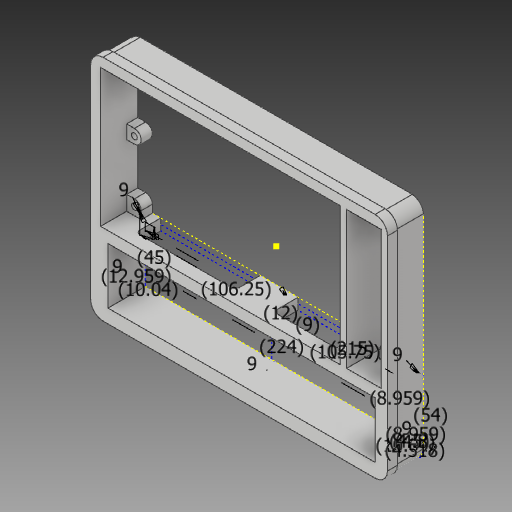
# Autodesk Inventor part: CyberDeckCover3
Saved by Autodesk Inventor 2019.4 (Build 234330000, 330)
## iProperties
Created: 2020-07-12
Part Number: CyberDeckCover3
Material: Generic
Document SubType Name: Modeling
Designer: Briti
Density: 1 g/cm^3
Appearance: Default
Author: Briti
Autodesk Inventor part; units mm, degrees
ref_plane "YZ Plane" through (0, 0, 0) normal (1, 0, 0) x (0, 1, 0)
ref_plane "XZ Plane" through (0, 0, 0) normal (0, 1, 0) x (-1, 0, 0)
ref_plane "XY Plane" through (0, 0, 0) normal (0, 0, 1) x (1, 0, 0)
sketch "Sketch1" plane through (0, 0, 0) normal (0, 0, 1) x (1, 0, 0)
  line L0 (-119.459, -91.9) -> (119.459, -91.9)
  line L1 (119.459, -91.9) -> (119.459, 91.9)
  line L2 (119.459, 91.9) -> (-119.459, 91.9)
  line L3 (-119.459, 91.9) -> (-119.459, -91.9)
  line L4 (-119.459, -91.9) -> (119.459, 91.9) construction
  line L5 (119.459, -91.9) -> (-119.459, 91.9) construction
  point P0 (0, 0)
  dimension "d0" = 238.918
  dimension "d1" = 183.8
  constraints: 12 end point, 2 midpoint, 2 parallel, 1 horizontal, 1 perpendicular
  measures "d0" distance of L2.end L1.end
  measures "d1" distance of L0.end L1.end
extrude "Extrusion1" add sketch "Sketch1" along normal blind 30
sketch "Sketch2" plane through (0, 0, 30) normal (0, 0, 1) x (1, 0, 0)
  arc A0 (-109.459, 91.9) -> (-119.459, 81.9) centre (-109.459, 81.9) ccw
  line L0 (119.459, 91.9) -> (-119.459, 91.9) projected
  line L1 (-119.459, 91.9) -> (-119.459, -91.9) projected
  line L2 (-119.459, 81.9) -> (-119.459, 91.9)
  line L3 (-109.459, 91.9) -> (-119.459, 91.9)
  arc A1 (-119.459, -81.9) -> (-109.459, -91.9) centre (-109.459, -81.9) ccw
  line L4 (-119.459, -91.9) -> (119.459, -91.9) projected
  line L5 (-119.459, -81.9) -> (-119.459, -91.9)
  line L6 (-109.459, -91.9) -> (-119.459, -91.9)
  arc A2 (109.459, -91.9) -> (119.459, -81.9) centre (109.459, -81.9) ccw
  line L7 (119.459, -91.9) -> (119.459, 91.9) projected
  line L8 (109.459, -91.9) -> (119.459, -91.9)
  line L9 (119.459, -81.9) -> (119.459, -91.9)
  arc A3 (119.459, 81.9) -> (109.459, 91.9) centre (109.459, 81.9) ccw
  line L10 (109.459, 91.9) -> (119.459, 91.9)
  line L11 (119.459, 81.9) -> (119.459, 91.9)
  point P0 (0, 0)
  dimension "d4" = 20
  dimension "d5" = 20
  dimension "d6" = 20
  dimension "d7" = 20
  constraints: 16 end point, 16 tangent, 8 point on circle, 8 point on line, 7 collinear, 4 centre point, 1 perpendicular
  measures "d4" diameter of A0
  measures "d5" diameter of A1
  measures "d6" diameter of A2
  measures "d7" diameter of A3
extrude "Extrusion2" add sketch "Sketch2" along normal blind 1 contours L0 A3 L7 A2 L4 A1 L1 A0
sketch "Sketch3" plane through (0, 0, 30) normal (0, 0, 1) x (1, 0, 0)
  line L0 (-119.459, -81.9) -> (-119.459, -91.9) projected
  arc A0 (-119.459, -81.9) -> (-109.459, -91.9) centre (-109.459, -81.9) ccw projected
  arc A1 (-119.459, -81.9) -> (-109.459, -91.9) centre (-109.459, -81.9) ccw
  line L1 (-119.459, -81.9) -> (-119.459, -91.9)
  line L2 (-119.459, -91.9) -> (-109.459, -91.9) projected
  line L3 (-109.459, -91.9) -> (-119.459, -91.9)
  arc A2 (-109.459, 91.9) -> (-119.459, 81.9) centre (-109.459, 81.9) ccw projected
  line L4 (-119.459, 81.9) -> (-119.459, -81.9) projected
  arc A3 (-109.459, 91.9) -> (-119.459, 81.9) centre (-109.459, 81.9) ccw
  line L5 (-119.459, 91.9) -> (-119.459, -91.9) projected
  line L6 (-119.459, 81.9) -> (-119.459, 91.9)
  line L7 (-119.459, 91.9) -> (-109.459, 91.9)
  arc A4 (119.459, 81.9) -> (109.459, 91.9) centre (109.459, 81.9) ccw projected
  arc A5 (119.459, 81.9) -> (109.459, 91.9) centre (109.459, 81.9) ccw
  line L8 (119.459, 81.9) -> (119.459, 91.9) projected
  line L9 (109.459, 91.9) -> (119.459, 91.9)
  line L10 (119.459, 91.9) -> (119.459, 81.9)
  arc A6 (109.459, -91.9) -> (119.459, -81.9) centre (109.459, -81.9) ccw projected
  arc A7 (109.459, -91.9) -> (119.459, -81.9) centre (109.459, -81.9) ccw
  line L11 (119.459, -91.9) -> (119.459, -81.9) projected
  line L12 (119.459, -81.9) -> (119.459, -91.9)
  line L13 (119.459, -91.9) -> (109.459, -91.9)
  point P0 (0, 0)
  constraints: 16 end point, 8 point on circle, 4 centre point, 3 collinear, 3 perpendicular, 3 tangent, 2 concentric, 1 horizontal, 1 vertical
extrude "Extrusion3" cut sketch "Sketch3" against normal blind 30
sketch "Sketch4" plane through (0, 0, 31) normal (0, 0, 1) x (1, 0, 0)
  line L0 (-111.459, -26.86) -> (81.501, -26.86)
  line L1 (81.501, -26.86) -> (81.501, 83.9)
  line L2 (81.501, 83.9) -> (-111.459, 83.9)
  line L3 (-111.459, 83.9) -> (-111.459, -26.86)
  line L4 (-111.459, -26.86) -> (81.501, 83.9) construction
  line L5 (81.501, -26.86) -> (-111.459, 83.9) construction
  line L6 (109.459, 91.9) -> (-109.459, 91.9) projected
  line L7 (-119.459, 81.9) -> (-119.459, -81.9) projected
  point P0 (0, 0)
  point P1 (-14.979, 28.52)
  dimension "d12" = 192.96
  dimension "d13" = 110.76
  dimension "d14" = 8
  dimension "d15" = 8
  constraints: 12 end point, 2 midpoint, 2 parallel, 1 horizontal, 1 perpendicular
  measures "d12" distance of L1.end L2.end
  measures "d13" distance of L0.end L1.end
  measures "d14" distance between parallel lines of L6 L2
  measures "d15" distance between parallel lines of L3 L7
extrude "Extrusion4" cut sketch "Sketch4" against normal blind 21
sketch "Sketch5" plane through (0, 0, 0) normal (0, 0, -1) x (-1, 0, 0)
  arc A0 (-109.459, 91.9) -> (-119.459, 81.9) centre (-109.459, 81.9) ccw projected
  arc A1 (-109.459, 91.9) -> (-119.459, 81.9) centre (-109.459, 81.9) ccw
  arc A2 (119.459, 81.9) -> (109.459, 91.9) centre (109.459, 81.9) ccw projected
  arc A3 (119.459, 81.9) -> (109.459, 91.9) centre (109.459, 81.9) ccw
  arc A4 (109.459, -91.9) -> (119.459, -81.9) centre (109.459, -81.9) ccw projected
  arc A5 (109.459, -91.9) -> (119.459, -81.9) centre (109.459, -81.9) ccw
  arc A6 (-119.459, -81.9) -> (-109.459, -91.9) centre (-109.459, -81.9) ccw projected
  arc A7 (-119.459, -81.9) -> (-109.459, -91.9) centre (-109.459, -81.9) ccw
  line L0 (-119.459, -91.9) -> (-119.459, 81.9) projected
  line L1 (-119.459, 81.9) -> (-119.459, -81.9)
  line L2 (109.459, -91.9) -> (-119.459, -91.9) projected
  line L3 (-109.459, -91.9) -> (109.459, -91.9)
  line L4 (119.459, 91.9) -> (119.459, -81.9) projected
  line L5 (119.459, -81.9) -> (119.459, 81.9)
  line L6 (-109.459, 91.9) -> (119.459, 91.9) projected
  line L7 (-109.459, 91.9) -> (109.459, 91.9)
  point P0 (0, 0)
  constraints: 8 end point, 8 point on circle, 4 centre point, 2 collinear, 2 tangent, 1 concentric, 1 horizontal, 1 vertical
extrude "Extrusion5" cut sketch "Sketch5" against normal blind 1 contours L6 A2 L4 A4 L2 A6 L0 A0
sketch "Sketch6" plane through (0, 0, 1) normal (0, 0, -1) x (-1, 0, 0)
  arc A0 (109.459, -91.9) -> (119.459, -81.9) centre (109.459, -81.9) ccw construction
  line L0 (119.459, -81.9) -> (118.459, -81.9) construction
  line L1 (109.459, -91.9) -> (109.459, -90.9) construction
  arc A1 (109.459, -90.9) -> (118.459, -81.9) centre (108.5046, -80.9456) ccw
  arc A2 (119.459, 81.9) -> (109.459, 91.9) centre (109.459, 81.9) ccw construction
  line L2 (119.459, 81.9) -> (118.459, 81.9) construction
  line L3 (109.459, 91.9) -> (109.459, 90.9) construction
  arc A3 (118.459, 81.9) -> (109.459, 90.9) centre (108.5046, 80.9456) ccw
  line L4 (119.459, 81.9) -> (119.459, -81.9) projected
  line L5 (118.459, 81.9) -> (118.459, -81.9)
  line L6 (-109.459, 91.9) -> (109.459, 91.9) construction
  line L7 (-109.459, 91.9) -> (-109.459, 90.9) construction
  line L8 (-119.459, 81.9) -> (-118.459, 81.9) construction
  arc A4 (-109.459, 90.9) -> (-118.459, 81.9) centre (-108.5046, 80.9456) ccw
  line L9 (-109.459, 90.9) -> (109.459, 90.9)
  arc A5 (-119.459, -81.9) -> (-109.459, -91.9) centre (-109.459, -81.9) ccw construction
  line L10 (-119.459, -81.9) -> (-118.459, -81.9) construction
  line L11 (109.459, -91.9) -> (-109.459, -91.9) construction
  line L12 (-109.459, -91.9) -> (-109.459, -90.9) construction
  arc A6 (-118.459, -81.9) -> (-109.459, -90.9) centre (-108.5046, -80.9456) ccw
  line L13 (-118.459, -81.9) -> (-118.459, 81.9)
  line L14 (-109.459, -90.9) -> (109.459, -90.9)
  arc A7 (-119.459, -81.9) -> (-109.459, -91.9) centre (-109.459, -81.9) ccw
  line L15 (-119.459, -81.9) -> (-119.459, 81.9) projected
  line L16 (-119.459, -81.9) -> (-119.459, 81.9)
  arc A8 (-109.459, 91.9) -> (-119.459, 81.9) centre (-109.459, 81.9) ccw
  line L17 (-109.459, 91.9) -> (109.459, 91.9)
  arc A9 (119.459, 81.9) -> (109.459, 91.9) centre (109.459, 81.9) ccw
  line L18 (119.459, 81.9) -> (119.459, -81.9)
  arc A10 (109.459, -91.9) -> (119.459, -81.9) centre (109.459, -81.9) ccw
  line L19 (109.459, -91.9) -> (-109.459, -91.9)
  point P0 (0, 0)
  dimension "d20" = 1
  dimension "d21" = 1
  dimension "d22" = 10
  dimension "d23" = 1
  dimension "d24" = 1
  dimension "d25" = 10
  dimension "d26" = 1
  dimension "d27" = 1
  dimension "d28" = 10
  dimension "d29" = 1
  dimension "d30" = 1
  dimension "d31" = 10
  constraints: 32 end point, 16 point on circle, 8 centre point, 5 vertical, 4 horizontal, 3 collinear, 3 concentric, 2 tangent
  measures "d20" distance of L0.start L0.end
  measures "d21" distance of L1.start L1.end
  measures "d22" radius of A1
  measures "d23" distance of L2.start L2.end
  measures "d24" distance of L3.start L3.end
  measures "d25" radius of A3
  measures "d26" distance of L6.start L7.end
  measures "d27" distance of L8.start L8.end
  measures "d28" radius of A4
  measures "d29" distance of L10.start L10.end
  measures "d30" distance of L11.end L12.end
  measures "d31" radius of A6
extrude "Extrusion6" cut sketch "Sketch6" against normal blind 22
sketch "Sketch8" plane through (0, 0, 10) normal (0, 0, 1) x (1, 0, 0)
  arc A0 (-105.209, 72.15) -> (-99.709, 77.65) centre (-105.209, 77.65) ccw
  line L0 (-111.459, 83.9) -> (81.501, 83.9) projected
  line L1 (-111.459, -26.86) -> (-111.459, 83.9) projected
  line L2 (-105.209, 77.65) -> (-99.709, 77.65) construction
  line L3 (-105.209, 77.65) -> (-105.209, 72.15) construction
  line L4 (-99.709, 77.65) -> (-99.709, 83.9)
  line L5 (-105.209, 72.15) -> (-111.459, 72.15)
  line L6 (-111.459, -26.86) -> (-111.459, 83.9) projected
  circle A1 centre (-105.209, 77.65) radius 2.4
  arc A2 (69.751, 77.65) -> (75.251, 72.15) centre (75.251, 77.65) ccw
  line L7 (81.501, 83.9) -> (81.501, -26.86) projected
  line L8 (75.251, 77.65) -> (75.251, 72.15) construction
  line L9 (75.251, 77.65) -> (69.751, 77.65) construction
  line L10 (69.751, 77.65) -> (69.751, 83.9)
  line L11 (75.251, 72.15) -> (81.501, 72.15)
  circle A3 centre (75.251, 77.65) radius 2.4
  arc A4 (75.251, -15.11) -> (69.751, -20.61) centre (75.251, -20.61) ccw
  line L12 (81.501, -26.86) -> (-111.459, -26.86) projected
  line L13 (75.251, -20.61) -> (75.251, -15.11) construction
  line L14 (75.251, -20.61) -> (69.751, -20.61) construction
  line L15 (75.251, -15.11) -> (81.501, -15.11)
  line L16 (69.751, -20.61) -> (69.751, -26.86)
  line L17 (81.501, -26.86) -> (-111.459, -26.86) projected
  circle A5 centre (75.251, -20.61) radius 2.4
  arc A6 (-99.709, -20.61) -> (-105.209, -15.11) centre (-105.209, -20.61) ccw
  line L18 (-105.209, -20.61) -> (-99.709, -20.61) construction
  line L19 (-105.209, -20.61) -> (-105.209, -15.11) construction
  line L20 (-105.209, -15.11) -> (-111.459, -15.11)
  line L21 (-99.709, -20.61) -> (-99.709, -26.86)
  circle A7 centre (-105.209, -20.61) radius 2.4
  arc A8 (-105.209, 23.02) -> (-105.209, 34.02) centre (-105.209, 28.52) ccw
  line L22 (-105.209, 28.52) -> (-105.209, 34.02) construction
  line L23 (-105.209, 28.52) -> (-105.209, 23.02) construction
  line L24 (-105.209, 34.02) -> (-111.459, 34.02)
  line L25 (-105.209, 23.02) -> (-111.459, 23.02)
  circle A9 centre (-105.209, 28.52) radius 2.4
  arc A10 (75.251, 34.02) -> (75.251, 23.02) centre (75.251, 28.52) ccw
  line L26 (75.251, 28.52) -> (75.251, 34.02) construction
  line L27 (75.251, 28.52) -> (75.251, 23.02) construction
  line L28 (75.251, 23.02) -> (81.501, 23.02)
  line L29 (75.251, 34.02) -> (81.501, 34.02)
  circle A11 centre (75.251, 28.52) radius 2.4
  line L30 (-99.709, 83.9) -> (69.751, 83.9)
  line L31 (81.501, 72.15) -> (81.501, 34.02)
  line L32 (81.501, -15.11) -> (81.501, 23.02)
  line L33 (69.751, -26.86) -> (-99.709, -26.86)
  line L34 (-111.459, -15.11) -> (-111.459, 23.02)
  line L35 (-111.459, 34.02) -> (-111.459, 72.15)
  line L36 (-111.459, 34.02) -> (-111.459, 23.02)
  line L37 (-111.459, 72.15) -> (-111.459, 83.9)
  line L38 (-99.709, 83.9) -> (-111.459, 83.9)
  line L39 (-111.459, -15.11) -> (-111.459, -26.86)
  line L40 (-111.459, -26.86) -> (-99.709, -26.86)
  line L41 (69.751, -26.86) -> (81.501, -26.86)
  line L42 (81.501, -15.11) -> (81.501, -26.86)
  line L43 (81.501, 23.02) -> (81.501, 34.02)
  line L44 (81.501, 72.15) -> (81.501, 83.9)
  line L45 (81.501, 83.9) -> (69.751, 83.9)
  line L46 (-14.979, 83.9) -> (-14.979, -26.86)
  point P0 (0, 0)
  dimension "d45" = 11
  dimension "d46" = 6.25
  dimension "d47" = 6.25
  dimension "d48" = 4.8
  dimension "d49" = 11
  dimension "d50" = 6.25
  dimension "d51" = 6.25
  dimension "d52" = 4.8
  dimension "d53" = 11
  dimension "d54" = 6.25
  dimension "d55" = 6.25
  dimension "d56" = 4.8
  dimension "d57" = 11
  dimension "d58" = 6.25
  dimension "d59" = 6.25
  dimension "d60" = 4.8
  dimension "d61" = 11
  dimension "d62" = 49.13
  dimension "d63" = 6.25
  dimension "d64" = 49.13
  dimension "d65" = 98.26
  dimension "d66" = 4.8
  dimension "d67" = 11
  dimension "d68" = 6.25
  dimension "d69" = 49.13
  dimension "d70" = 4.8
  dimension "d71" = 49.13
  constraints: 82 end point, 24 perpendicular, 14 point on line, 12 centre point, 12 point on circle, 10 tangent, 8 collinear, 6 coincident, 4 vertical, 2 horizontal, 2 midpoint
  measures "d45" diameter of A0
  measures "d46" distance from line of L0 L2.start
  measures "d47" distance from line of L1 L2.start
  measures "d48" diameter of A1
  measures "d49" diameter of A2
  measures "d50" distance from line of L0 L8.start
  measures "d51" distance from line of L8.start L7
  measures "d52" diameter of A3
  measures "d53" diameter of A4
  measures "d54" distance from line of L7 L13.start
  measures "d55" distance from line of L13.start L12
  measures "d56" diameter of A5
  measures "d57" diameter of A6
  measures "d58" distance from line of L1 L18.start
  measures "d59" distance from line of L18.start L12
  measures "d60" diameter of A7
  measures "d61" diameter of A8
  measures "d62" distance of L2.start L22.start
  measures "d63" distance from line of L1 L22.start
  measures "d64" distance of L18.start L22.start
  measures "d65" distance of A7.centre L2.start
  measures "d66" diameter of A9
  measures "d67" diameter of A10
  measures "d68" distance from line of L7 L26.start
  measures "d69" distance of L26.start L8.start
  measures "d70" diameter of A11
  measures "d71" distance of L13.start L26.start
extrude "Extrusion7" cut sketch "Sketch8" against normal blind 10 contours A0 L4 L0 L46 L12 L21 A6 L20 L1 L25 A8 L24 L5 | L0 L10 A2 L11 L7 L29 A10 L28 L15 A4 L16 L12 L46
sketch "Sketch9" plane through (0, 0, 10) normal (0, 0, 1) x (1, 0, 0)
  arc A0 (-105.209, 23.02) -> (-105.209, 34.02) centre (-105.209, 28.52) ccw projected
  circle A1 centre (-105.209, 28.52) radius 2.4
  arc A2 (-105.209, 72.15) -> (-99.709, 77.65) centre (-105.209, 77.65) ccw projected
  circle A3 centre (-105.209, 77.65) radius 2.4
  arc A4 (-99.709, -20.61) -> (-105.209, -15.11) centre (-105.209, -20.61) ccw projected
  circle A5 centre (-105.209, -20.61) radius 2.4
  arc A6 (75.251, -15.11) -> (69.751, -20.61) centre (75.251, -20.61) ccw projected
  circle A7 centre (75.251, -20.61) radius 2.4
  arc A8 (75.251, 34.02) -> (75.251, 23.02) centre (75.251, 28.52) ccw projected
  circle A9 centre (75.251, 28.52) radius 2.4
  arc A10 (69.751, 77.65) -> (75.251, 72.15) centre (75.251, 77.65) ccw projected
  circle A11 centre (75.251, 77.65) radius 2.4
  point P0 (0, 0)
  dimension "d74" = 4.8
  dimension "d75" = 4.8
  dimension "d76" = 4.8
  dimension "d77" = 4.8
  dimension "d78" = 4.8
  dimension "d79" = 4.8
  constraints: 6 centre point, 6 coincident
  measures "d74" diameter of A1
  measures "d75" diameter of A3
  measures "d76" diameter of A5
  measures "d77" diameter of A7
  measures "d78" diameter of A9
  measures "d79" diameter of A11
extrude "Extrusion8" cut sketch "Sketch9" against normal blind 10
sketch "Sketch10" plane through (0, 0, 31) normal (0, 0, 1) x (1, 0, 0)
  line L0 (-105.5, -35.86) -> (109.5, -35.86)
  line L1 (109.5, -35.86) -> (109.5, -80.86)
  line L2 (109.5, -80.86) -> (-105.5, -80.86)
  line L3 (-105.5, -80.86) -> (-105.5, -35.86)
  line L4 (81.501, -26.86) -> (-111.459, -26.86) projected
  line L5 (-109.459, -91.9) -> (109.459, -91.9) projected
  line L6 (-119.459, 81.9) -> (-119.459, -81.9) projected
  line L7 (119.459, -81.9) -> (119.459, 81.9) projected
  point P0 (0, 0)
  dimension "d82" = 215
  dimension "d83" = 45
  dimension "d84" = 9
  dimension "d85" = 11.04
  dimension "d86" = 13.959
  dimension "d87" = 9.959
  constraints: 8 end point, 2 parallel, 1 horizontal, 1 perpendicular
  measures "d82" distance of L0.start L0.end
  measures "d83" distance of L0.end L1.end
  measures "d84" distance between parallel lines of L0 L4
  measures "d85" distance between parallel lines of L5 L2
  measures "d86" distance between parallel lines of L6 L3
  measures "d87" distance between parallel lines of L7 L1
extrude "Extrusion9" cut sketch "Sketch10" against normal blind 30
sketch "Sketch11" plane through (0, 0, 1) normal (0, 0, -1) x (-1, 0, 0)
  line L0 (-109.5, -35.86) -> (105.5, -35.86) construction
  line L1 (-109.5, -35.86) -> (-69.5, -35.86) construction
  line L2 (99.709, -26.86) -> (-69.751, -26.86) projected
  line L3 (-69.5, -35.86) -> (-17.5, -35.86)
  line L4 (-17.5, -35.86) -> (-17.5, -26.86)
  line L5 (-17.5, -26.86) -> (-69.5, -26.86)
  line L6 (-69.5, -26.86) -> (-69.5, -35.86)
  line L7 (-17.5, -26.86) -> (13, -26.86)
  line L8 (13, -26.86) -> (13, -35.86)
  line L9 (13, -35.86) -> (-17.5, -35.86)
  line L10 (-17.5, -35.86) -> (-17.5, -26.86)
  line L11 (13, -26.86) -> (93, -26.86)
  line L12 (93, -26.86) -> (93, -35.86)
  line L13 (93, -35.86) -> (13, -35.86)
  line L14 (13, -35.86) -> (13, -26.86)
  line L15 (-17.5, -31.36) -> (13, -31.36) construction
  circle A0 centre (-8.25, -31.36) radius 2.4
  circle A1 centre (3.75, -31.36) radius 2.4
  line L16 (-109.5, -35.86) -> (-109.5, -26.86) construction
  line L17 (-109.5, -26.86) -> (-118.459, -26.86) construction
  line L18 (-118.459, 81.9) -> (-118.459, -81.9) construction
  line L19 (-109.5, -35.86) -> (-122.459, -35.86) construction
  circle A2 centre (-114, -31.36) radius 2.4
  line L20 (-109.5, -80.86) -> (-109.5, -35.86) projected
  circle A3 centre (-114, -85.36) radius 2.4
  line L21 (105.5, -80.86) -> (-109.5, -80.86) projected
  circle A4 centre (110, -31.36) radius 2.4
  line L22 (105.5, -35.86) -> (105.5, -80.86) projected
  circle A5 centre (110, -85.36) radius 2.4
  line L23 (110, -85.36) -> (-114, -85.36) construction
  line L24 (-8.25, -31.36) -> (-8.25, -85.36) construction
  line L25 (3.75, -31.36) -> (3.75, -85.36) construction
  circle A6 centre (-8.25, -85.36) radius 2.4
  circle A7 centre (3.75, -85.36) radius 2.4
  point P0 (0, 0)
  dimension "d90" = 40
  dimension "d91" = 52
  dimension "d92" = 30.5
  dimension "d93" = 80
  dimension "d94" = 4.8
  dimension "d95" = 4.8
  dimension "d96" = 9.25
  dimension "d97" = 9.25
  dimension "d98" = 12
  dimension "d120" = 4.5
  dimension "d121" = 9
  dimension "d122" = 4.8
  dimension "d123" = 4.5
  dimension "d124" = 4.5
  dimension "d125" = 4.8
  dimension "d126" = 4.5
  dimension "d127" = 4.5
  dimension "d128" = 4.8
  dimension "d129" = 4.5
  dimension "d130" = 4.5
  dimension "d131" = 4.8
  dimension "d132" = 4.5
  dimension "d133" = 4.5
  dimension "d134" = 4.8
  dimension "d135" = 4.8
  constraints: 40 end point, 9 point on line, 8 centre point, 6 parallel, 6 perpendicular, 4 horizontal, 2 coincident, 2 midpoint, 1 vertical
  measures "d90" distance of L0.start L1.end
  measures "d91" distance of L5.end L4.end
  measures "d92" distance of L8.end L9.end
  measures "d93" distance of L12.end L13.end
  measures "d94" diameter of A0
  measures "d95" diameter of A1
  measures "d96" distance from line of L4 L24.start
  measures "d97" distance from line of L8 L25.start
  measures "d98" distance of L25.start L24.start
  measures "d120" distance from line of L7 L25.start
  measures "d121" distance of L0.start L16.end
  measures "d122" diameter of A2
  measures "d123" distance from line of L0 A2.centre
  measures "d124" distance from line of L20 A2.centre
  measures "d125" diameter of A3
  measures "d126" distance from line of L21 L23.end
  measures "d127" distance from line of L20 L23.end
  measures "d128" diameter of A4
  measures "d129" distance from line of L0 A4.centre
  measures "d130" distance from line of L22 A4.centre
  measures "d131" diameter of A5
  measures "d132" distance from line of L23.start L22
  measures "d133" distance from line of L21 L23.start
  measures "d134" diameter of A6
  measures "d135" diameter of A7
extrude "Extrusion10" cut sketch "Sketch11" against normal blind 20 contours A0 | A1 | A2 | A3 | A4 | A5 | A6 | A7
sketch "Sketch12" plane through (-105.5, -35.86, 31) normal (0, -1, 0) x (1, 0, 0)
  line L0 (215, -30) -> (0, -30) construction
  line L1 (215, -30) -> (175, -30) construction
  line L2 (175.251, -21) -> (175.251, -30) construction
  line L3 (175, -30) -> (123, -30)
  line L4 (123, -30) -> (123, -13)
  line L5 (126, -10) -> (172, -10)
  line L6 (175, -13) -> (175, -30)
  line L7 (123, -30) -> (92.5, -30)
  line L8 (92.5, -30) -> (92.5, -13)
  line L9 (92.5, -10) -> (123, -10)
  line L10 (123, -13) -> (123, -30)
  line L11 (89.5, -10) -> (15.5, -10)
  line L12 (12.5, -13) -> (12.5, -30)
  line L13 (12.5, -30) -> (92.5, -30)
  line L14 (92.5, -30) -> (92.5, -13)
  line L15 (0, 0) -> (215, 0) projected
  arc A0 (175, -13) -> (172, -10) centre (172, -13) ccw
  arc A1 (126, -10) -> (123, -13) centre (126, -13) ccw
  arc A2 (92.5, -13) -> (89.5, -10) centre (89.5, -13) ccw
  line L16 (92.5, -10) -> (89.5, -10) construction
  arc A3 (15.5, -10) -> (12.5, -13) centre (15.5, -13) ccw
  point P0 (105.5, -31)
  dimension "d101" = 40
  dimension "d102" = 52
  dimension "d103" = 30.5
  dimension "d104" = 80
  dimension "d105" = 10
  dimension "d106" = 6
  dimension "d107" = 6
  dimension "d108" = 6
  dimension "d109" = 10
  dimension "d110" = 6
  constraints: 28 end point, 8 point on circle, 8 tangent, 6 parallel, 4 centre point, 4 perpendicular, 3 horizontal, 2 point on line
  measures "d101" distance of L0.start L1.end
  measures "d102" distance of L4.end L6.start
  measures "d103" distance of L9.start L9.end
  measures "d104" distance of L13.end L12.end
  measures "d105" distance between parallel lines of L15 L5
  measures "d106" diameter of A0
  measures "d107" diameter of A1
  measures "d108" diameter of A2
  measures "d109" distance between parallel lines of L15 L11
  measures "d110" diameter of A3
extrude "Extrusion11" cut sketch "Sketch12" against normal blind 20
sketch "Sketch17" plane through (0, 0, 31) normal (0, 0, 1) x (1, 0, 0)
  line L0 (86.501, -26.86) -> (114.459, -26.86)
  line L1 (114.459, -26.86) -> (114.459, 83.9)
  line L2 (114.459, 83.9) -> (86.501, 83.9)
  line L3 (86.501, 83.9) -> (86.501, -26.86)
  line L4 (81.501, 83.9) -> (81.501, -26.86) projected
  line L5 (119.459, -81.9) -> (119.459, 81.9) projected
  line L6 (109.459, 91.9) -> (-109.459, 91.9) projected
  line L7 (-105.5, -35.86) -> (109.5, -35.86) projected
  point P0 (0, 0)
  dimension "d148" = 5
  dimension "d149" = 5
  dimension "d150" = 8
  dimension "d151" = 9
  dimension "d167" = 27.958
  dimension "d168" = 110.76
  constraints: 8 end point, 2 parallel, 1 horizontal, 1 perpendicular
  measures "d148" distance between parallel lines of L3 L4
  measures "d149" distance between parallel lines of L5 L1
  measures "d150" distance between parallel lines of L2 L6
  measures "d151" distance between parallel lines of L7 L0
  measures "d167" distance of L0.start L0.end
  measures "d168" distance of L0.end L1.end
extrude "Extrusion14" cut sketch "Sketch17" against normal blind 20
sketch "Sketch18" plane through (0, 0, 11) normal (0, 0, 1) x (1, 0, 0)
  line L0 (114.459, -26.86) -> (86.501, -26.86) construction
  line L1 (100.48, -26.86) -> (100.48, -21.36) construction
  arc A0 (107.98, -21.36) -> (92.98, -21.36) centre (100.48, -21.36) ccw
  line L2 (107.98, -21.36) -> (107.98, -26.86)
  line L3 (92.98, -21.36) -> (92.98, -26.86)
  line L4 (86.501, 83.9) -> (114.459, 83.9) construction
  line L5 (100.48, 83.9) -> (100.48, 78.4) construction
  arc A1 (94.98, 78.4) -> (105.98, 78.4) centre (100.48, 78.4) ccw
  line L6 (105.98, 78.4) -> (105.98, 83.9)
  line L7 (94.98, 78.4) -> (94.98, 83.9)
  line L8 (94.98, 83.9) -> (86.501, 83.9)
  line L9 (86.501, 83.9) -> (86.501, -26.86)
  line L10 (92.98, -26.86) -> (86.501, -26.86)
  line L11 (114.459, 83.9) -> (114.459, -26.86) projected
  line L12 (107.98, -26.86) -> (114.459, -26.86)
  line L13 (114.459, -26.86) -> (114.459, 83.9)
  line L14 (114.459, 83.9) -> (105.98, 83.9)
  point P0 (0, 0)
  dimension "d154" = 5.5
  dimension "d155" = 5.5
  constraints: 24 end point, 6 perpendicular, 4 point on circle, 4 point on line, 3 tangent, 2 centre point, 2 coincident, 2 collinear, 2 horizontal, 2 midpoint, 2 vertical
  measures "d154" distance of L1.start L1.end
  measures "d155" distance of L5.start L5.end
extrude "Extrusion15" cut sketch "Sketch18" against normal blind 10
sketch "Sketch19" plane through (0, 0, 11) normal (0, 0, 1) x (1, 0, 0)
  arc A0 (107.98, -21.36) -> (92.98, -21.36) centre (100.48, -21.36) ccw projected
  circle A1 centre (100.48, -21.36) radius 2.4
  arc A2 (94.98, 78.4) -> (105.98, 78.4) centre (100.48, 78.4) ccw projected
  circle A3 centre (100.48, 78.4) radius 2.4
  line L0 (100.48, -21.36) -> (100.48, 78.4) construction
  line L1 (100.48, -21.36) -> (114.459, -21.36) construction
  line L2 (114.459, 83.9) -> (114.459, -26.86) construction
  line L3 (86.501, 83.9) -> (114.459, 83.9) construction
  line L4 (114.459, 83.9) -> (114.459, -26.86) construction
  point P0 (0, 0)
  dimension "d158" = 4.8
  dimension "d159" = 4.8
  dimension "d164" = 99.76
  dimension "d165" = 13.979
  dimension "d166" = 110.76
  constraints: 6 end point, 2 centre point, 2 coincident, 1 horizontal, 1 perpendicular, 1 point on line, 1 vertical
  measures "d158" diameter of A1
  measures "d159" diameter of A3
  measures "d164" distance of L0.start L0.end
  measures "d165" distance of L0.start L1.end
  measures "d166" distance of L2.start L2.end
extrude "Extrusion16" cut sketch "Sketch19" against normal blind 10
sketch "Sketch22" plane through (0, 0, 1) normal (0, 0, -1) x (-1, 0, 0)
  circle A0 centre (-8.25, -31.36) radius 2.4 construction
  circle A1 centre (3.75, -31.36) radius 2.4 construction
  line L0 (-8.25, -31.36) -> (3.75, -31.36) construction
  circle A2 centre (-8.25, -85.36) radius 2.4 construction
  circle A3 centre (3.75, -85.36) radius 2.4 construction
  line L1 (-8.25, -85.36) -> (3.75, -85.36) construction
  line L2 (3.75, -85.36) -> (3.75, -31.36) construction
  circle A4 centre (110, -85.36) radius 2.4 construction
  circle A5 centre (-114, -85.36) radius 2.4 construction
  line L3 (110, -85.36) -> (-114, -85.36) construction
  circle A6 centre (-114, -31.36) radius 2.4 construction
  line L4 (-114, -85.36) -> (-114, -31.36) construction
  line L5 (-114, -31.36) -> (-8.25, -31.36) construction
  circle A7 centre (110, -31.36) radius 2.4 construction
  line L6 (3.75, -31.36) -> (110, -31.36) construction
  circle A8 centre (-8.25, -31.36) radius 4.5 construction
  line L7 (-81.501, -26.86) -> (111.459, -26.86) construction
  circle A9 centre (110, -31.36) radius 4.5 construction
  circle A10 centre (-114, -31.36) radius 4.5 construction
  circle A11 centre (3.75, -85.36) radius 4.5 construction
  line L8 (-118.459, 81.9) -> (-118.459, -81.9) construction
  arc A12 (-118.459, -81.9) -> (-109.459, -90.9) centre (-108.5046, -80.9456) ccw construction
  arc A13 (-118.459, -81.9) -> (-109.459, -90.9) centre (-108.5046, -80.9456) ccw construction
  line L9 (-109.5, -80.86) -> (-109.5, -35.86) construction
  line L10 (109.459, -91.9) -> (-109.459, -91.9) construction
  line L11 (-109.5, -80.86) -> (-109.459, -90.9) construction
  circle A14 centre (110, -85.36) radius 4.5 construction
  line L12 (114.5, -85.36) -> (114.5, -31.36) construction
  line L13 (-109.4816, -85.36) -> (-114, -85.36) construction
  line L14 (-109.4816, -85.36) -> (-114, -85.36) construction
  line L15 (105.5, -35.86) -> (-109.5, -35.86) construction
  line L16 (105.5, -35.86) -> (-109.5, -35.86) construction
  line L17 (-109.5, -80.86) -> (105.5, -80.86) construction
  line L18 (105.5, -35.86) -> (105.5, -80.86) construction
  arc A15 (-118.459, -81.0246) -> (-109.459, -90.9) centre (-108.541, -81.0246) ccw construction
  line L19 (105.5, -80.86) -> (105.5, -90.9) construction
  line L20 (-109.459, -90.9) -> (109.459, -90.9) construction
  line L21 (105.5, -80.86) -> (118.459, -80.86) construction
  line L22 (118.459, -81.9) -> (118.459, 81.9) construction
  line L23 (118.459, -80.86) -> (118.459, -81.9) construction
  line L24 (105.5, -90.9) -> (109.459, -90.9) construction
  arc A16 (109.459, -90.9) -> (118.459, -81.9) centre (108.5046, -80.9456) ccw construction
  line L25 (118.459, -80.86) -> (118.459, -81.9) construction
  circle A17 centre (-114, -85.36) radius 4.5 construction
  line L26 (-109.5, -80.86) -> (-114, -80.86) construction
  point P0 (0, 0)
  dimension "d175" = 9
  dimension "d178" = 9
  dimension "d190" = 9
  dimension "d170" = 106.25
  dimension "d171" = 12
  dimension "d172" = 105.75
  dimension "d173" = 54
  dimension "d174" = 224
  dimension "d176" = 9
  dimension "d177" = 9
  dimension "d179" = 4.5
  dimension "d180" = 4.5184
  dimension "d181" = 9
  dimension "d182" = 215
  dimension "d183" = 45
  dimension "d184" = 8.959
  dimension "d185" = 4.8
  dimension "d186" = 10.04
  dimension "d187" = 8.959
  dimension "d188" = 10.04
  dimension "d189" = 12.959
  constraints: 38 end point, 6 coincident, 6 point on line, 5 centre point, 5 collinear, 5 perpendicular, 4 horizontal, 4 point on circle, 4 vertical, 2 horizontal alignment, 2 tangent, 1 concentric, 1 vertical alignment, 6 other
  measures "d170" distance of L0.end L6.end
  measures "d171" distance of L0.start L0.end
  measures "d172" distance of L4.end L0.start
  measures "d173" distance of L3.end L4.end
  measures "d174" distance of L3.start L3.end
  measures "d176" diameter of A10
  measures "d177" diameter of A11
  measures "d179" vertical distance of L13.start L9.start
  measures "d180" distance of L13.start L3.end
  measures "d181" diameter of A8
  measures "d182" distance of L15.start L9.end
  measures "d183" distance of L15.start L17.end
  measures "d184" distance between parallel lines of L9 L8
  measures "d185" diameter of A5
  measures "d186" vertical distance of L11.end L9.start
  measures "d187" horizontal distance of A15.start L9.start
  measures "d188" distance of L17.end L19.end
  measures "d189" distance of L17.end L21.end
body "Solid1"
